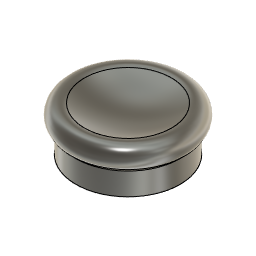
Topper - concave v2 (Autodesk Fusion 360 design; units mm, degrees)
Autodesk Fusion 360 part; units mm, degrees
sketch "Sketch1" plane through (0, 0, 0) normal (0, 1, 0) x (1, 0, 0)
  line L0 (0, 0) -> (7, 0)
  line L1 (7, 0) -> (7, -3)
  line L2 (7, -3) -> (7.5607, -3.5607)
  arc A0 (5.8427, -5.9696) -> (0, -4.6213) centre (0, -17.9547) ccw
  line L3 (0, -4.6213) -> (0, 0)
  arc A1 (5.8427, -5.9696) -> (7.5607, -3.5607) centre (6.5, -4.6213) ccw
  line L4 (0, -4.6213) -> (4, -4.6213) construction
  line L5 (0, -6.1213) -> (12, -6.1213) construction
  line L6 (8, -7.8142) -> (8, 1) construction
  dimension "d1" = 7
  dimension "d2" = 3
  dimension "d3" = 1.5
  dimension "d4" = 1.5
  dimension "d6" = 8
  dimension "d7" = 45
  constraint coincident L0.start L3.end
  constraint horizontal L0
  constraint perpendicular L0 L1
  constraint perpendicular L0 L3
  constraint tangent A0 A1
  constraint tangent L2 A1
  constraint perpendicular L3 L4
  constraint tangent A0 L4
  constraint horizontal L5
  constraint tangent A1 L5
  constraint perpendicular L5 L6
  constraint tangent A1 L6
  measures "d1" distance of L0.start L0.end
  measures "d2" distance of L0.end L1.end
  measures "d3" radius of A1
  measures "d4" distance of L4 L5
  measures "d6" distance of L3 L6
  measures "d7" angle of L2 L5
revolve "Revolve1" add sketch "Sketch1" angle 360 about axis through (0, 0, 4.6213) along (0, 0, -1)
sketch "Sketch2" plane through (0, 0, 0) normal (0, 0, -1) x (1, 0, 0)
  circle A0 centre (0, 0) radius 7
  line L0 (1.55, 1.05) -> (1.55, -1.05)
  line L1 (0.55, 2.05) -> (-0.55, 2.05)
  line L2 (-1.55, 1.05) -> (-1.55, -1.05)
  arc A1 (0.55, -2.05) -> (1.55, -1.05) centre (0.55, -1.05) ccw
  arc A2 (1.55, 1.05) -> (0.55, 2.05) centre (0.55, 1.05) ccw
  arc A3 (-0.55, 2.05) -> (-1.55, 1.05) centre (-0.55, 1.05) ccw
  line L3 (0.55, -2.05) -> (-0.55, -2.05)
  arc A4 (-1.55, -1.05) -> (-0.55, -2.05) centre (-0.55, -1.05) ccw
  point P0 (1.55, 2.05)
  point P1 (1.55, 0)
  point P2 (0, -2.05)
  point P3 (-1.55, 2.05)
  point P4 (1.55, -2.05)
  dimension "d11" = 4.1
  dimension "d12" = 3.1
  dimension "d13" = 1
  constraint vertical L2
  constraint vertical L0
  constraint horizontal P1 A0.centre
  constraint coincident A0.centre origin
  constraint horizontal L3
  constraint horizontal L1
  constraint vertical A0.centre P2
  constraint coincident P2 L3
  constraint coincident P1 L0
  constraint coincident P4 L3
  constraint coincident P4 L0
  constraint tangent A1 L3
  constraint tangent L0 A1
  constraint coincident P3 L1
  constraint coincident P3 L2
  constraint tangent L1 A3
  constraint tangent L2 A3
  constraint equal A1 A3
  constraint tangent L3 A4
  constraint tangent L2 A4
  constraint equal A1 A4
  constraint coincident P0 L0
  constraint coincident P0 L1
  constraint tangent L0 A2
  constraint tangent L1 A2
  constraint equal A1 A2
  constraint midpoint P2 L3
  constraint midpoint P1 L0
  measures "d11" distance of P0 P4
  measures "d12" distance of P0 P3
  measures "d13" radius of A1
extrude "Extrude1" cut sketch "Sketch2" against normal blind 2.5 contours L0 L1 L2 A1 A2 A3 L3 A4
